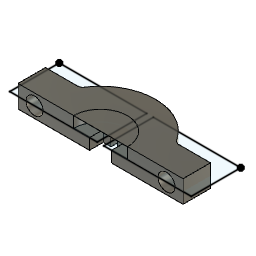
holder_clamp v2 (Autodesk Fusion 360 design; units mm, degrees)
Autodesk Fusion 360 part; units mm, degrees
sketch "スケッチ1" plane through (0, 0, 0) normal (0, 0, 1) x (1, 0, 0)
  line L0 (-16.5, 22) -> (16.5, 22)
  line L1 (16.5, 22) -> (16.5, 0)
  line L2 (16.5, 0) -> (-16.5, 0)
  line L3 (-16.5, 0) -> (-16.5, 22)
  dimension "d7" = 22
  dimension "d8" = 33
  constraint horizontal L0
  constraint vertical L1
  constraint horizontal L2
  constraint vertical L3
  constraint coincident origin L2
  constraint midpoint origin L2
  measures "d7" distance of L0.end L1.end
  measures "d8" distance of L0.start L0.end
extrude "押し出し1" add sketch "スケッチ1" along normal blind 2
sketch "スケッチ3" plane through (0, 0, 0) normal (0, 0, -1) x (1, 0, 0)
  line L0 (16.5, 0) -> (-16.5, 0)
  line L1 (-16.5, 0) -> (-16.5, -22)
  line L2 (-16.5, -22) -> (16.5, -22)
  line L3 (16.5, -22) -> (16.5, 0)
  arc A0 (-4.9, -13) -> (4.9, -13) centre (0, -13) ccw
  line L4 (16.5, -13) -> (-16.5, -13)
  dimension "d9" = 9.8
  dimension "d10" = 9
  constraint coincident L3 L4.start
  constraint coincident L1 L4.end
  constraint perpendicular L1 L4
  constraint coincident A0.centre L4
  measures "d9" diameter of A0
  measures "d10" distance of L2 A0.centre
extrude "押し出し2" add sketch "スケッチ3" along normal blind 2 contours L1 L2 L3 A0 L4
sketch "スケッチ4" plane through (0, 0, -2) normal (0, 0, -1) x (1, 0, 0)
  line L0 (-4.9, -13) -> (-16.5, -13)
  line L1 (-16.5, -13) -> (-16.5, -22)
  line L2 (-16.5, -22) -> (16.5, -22)
  line L3 (16.5, -22) -> (16.5, -13)
  line L4 (16.5, -13) -> (4.9, -13)
  arc A0 (-4.9, -13) -> (4.9, -13) centre (0, -13) ccw
  line L5 (16.5, -22) -> (0.6, -22)
  line L6 (0.6, -22) -> (0.6, -13)
  line L7 (0.6, -13) -> (16.5, -13)
  line L8 (16.5, -13) -> (16.5, -22)
  line L9 (-16.5, -22) -> (-0.6, -22)
  line L10 (-0.6, -22) -> (-0.6, -13)
  line L11 (-0.6, -13) -> (-16.5, -13)
  line L12 (-16.5, -13) -> (-16.5, -22)
  dimension "d13" = 1.2
  constraint horizontal L5
  constraint vertical L6
  constraint horizontal L7
  constraint vertical L8
  constraint coincident L2.end L3.start
  constraint horizontal L9
  constraint vertical L10
  constraint horizontal L11
  constraint vertical L12
  constraint coincident L1.end L2.start
  constraint equal L5 L9
  constraint equal L8 L12
  constraint equal L1 L12
  measures "d13" distance of L6 L10
extrude "押し出し3" add sketch "スケッチ4" along normal blind 2
sketch "スケッチ5" plane through (0, 0, 0) normal (0, 0, -1) x (1, 0, 0)
  line L0 (4.9, -13) -> (16.5, -13)
  line L1 (16.5, -13) -> (16.5, 0)
  line L2 (16.5, 0) -> (-16.5, 0)
  line L3 (-16.5, 0) -> (-16.5, -13)
  line L4 (-16.5, -13) -> (-4.9, -13)
  arc A0 (-4.9, -13) -> (4.9, -13) centre (0, -13) ccw
  line L5 (-3.75, 0) -> (3.75, 0)
  line L6 (3.75, 0) -> (3.75, -18)
  line L7 (3.75, -18) -> (-3.75, -18)
  line L8 (-3.75, -18) -> (-3.75, 0)
  line L9 (0, -1.75) -> (0, -22.5)
  line L10 (3.75, -7) -> (16.5, -7)
  line L11 (-3.75, -7) -> (-16.5, -7)
  dimension "d17" = 7.5
  dimension "d18" = 11
  dimension "d19" = 11
  constraint horizontal L5
  constraint vertical L6
  constraint horizontal L7
  constraint vertical L8
  constraint coincident L2 L5.start
  constraint symmetric L6 L8 L9
  constraint coincident L6 L10.start
  constraint perpendicular L6 L10
  constraint coincident L1 L10.end
  constraint coincident L8 L11.start
  constraint coincident L3 L11.end
  constraint perpendicular L3 L11
  measures "d17" distance of L5.start L5.end
  measures "d18" distance of L6.end L10.start
  measures "d19" distance of L7.end L11.start
sketch "スケッチ9" plane through (0, 13, 0) normal (0, -1, 0) x (1, 0, 0)
  line L0 (-4.9, 0) -> (-16.5, 0)
  line L1 (-16.5, 0) -> (-16.5, -4)
  line L2 (-16.5, -4) -> (-0.6, -4)
  line L3 (-0.6, -4) -> (-0.6, -2)
  line L4 (-0.6, -2) -> (-4.9, -2)
  line L5 (-4.9, -2) -> (-4.9, 0)
  line L6 (-2, -2) -> (2, -2)
  line L7 (2, -2) -> (2, -4)
  line L8 (2, -4) -> (-2, -4)
  line L9 (-2, -4) -> (-2, -2)
  line L10 (16.5, -4) -> (0.6, -4)
  dimension "d37" = 4
  dimension "d38" = 2
  constraint horizontal L6
  constraint vertical L7
  constraint horizontal L8
  constraint vertical L9
  constraint coincident L4 L6.start
  constraint collinear L8 L10
  measures "d37" distance of L7.end L8.end
  measures "d38" distance of origin L7
extrude "押し出し7" cut sketch "スケッチ9" against normal blind 2.5 contours L2 L3 L4 L6 L8 L9 | L3 L6 L7 L8 L10
sketch "スケッチ11" plane through (0, 22, 0) normal (0, 1, 0) x (-1, 0, 0)
  line L0 (16.5, -4) -> (16.5, 2)
  line L1 (16.5, 2) -> (-16.5, 2)
  line L2 (-16.5, 2) -> (-16.5, -4)
  line L3 (-16.5, -4) -> (16.5, -4)
  line L4 (16.5, 2) -> (-13.5, 2)
  line L5 (-13.5, 2) -> (-13.5, 12)
  line L6 (-13.5, 12) -> (16.5, 12)
  line L7 (16.5, 12) -> (16.5, 2)
  dimension "d49" = 10
  constraint horizontal L4
  constraint vertical L5
  constraint horizontal L6
  constraint vertical L7
  constraint coincident L0.end L1.start
  measures "d49" distance of L0.end L6.end
ref_plane "作業平面1" through (0, 11, -1) normal (0, 1, 0) x (-1, 0, 0)
sketch "スケッチ13" plane through (0, 11, -1) normal (0, 1, 0) x (1, 0, 0)
  line L0 (16.5, -10) -> (-16.5, -10)
  line L1 (-16.5, -10) -> (-16.5, -3)
  line L2 (-16.5, -3) -> (16.5, -3)
  line L3 (16.5, -3) -> (16.5, -10)
  line L4 (16.5, 3) -> (16.5, -3)
  line L5 (-16.5, 3) -> (-16.5, -3)
  circle A0 centre (0, -6.5) radius 2.25
  dimension "d53" = 7
  dimension "d54" = 4.5
  dimension "d58" = 3.5
  constraint horizontal L0
  constraint vertical L1
  constraint horizontal L2
  constraint vertical L3
  constraint collinear L3 L4
  constraint coincident L2 L1.end
  measures "d53" distance of L0.end L1.end
  measures "d54" diameter of A0
  measures "d58" distance of L2 A0.centre
extrude "押し出し11" add sketch "スケッチ13" along normal blind -2 and the other way blind -8
sketch "Sketch17" plane through (16.5, 0, 0) normal (1, 0, 0) x (0, 1, 0)
  line L0 (22, -4) -> (22, 2)
  line L1 (22, 2) -> (19, 2)
  line L2 (19, 2) -> (19, 9)
  line L3 (19, 9) -> (9, 9)
  line L4 (9, 9) -> (9, 2)
  line L5 (9, 2) -> (0, 2)
  line L6 (0, 2) -> (0, 0)
  line L7 (0, 0) -> (13, 0)
  line L8 (13, 0) -> (13, -4)
  line L9 (13, -4) -> (22, -4)
  line L10 (11, 9) -> (17, 9)
  line L11 (17, 9) -> (17, 2)
  line L12 (17, 2) -> (11, 2)
  line L13 (11, 2) -> (11, 9)
  constraint horizontal L10
  constraint vertical L11
  constraint horizontal L12
  constraint vertical L13
  constraint coincident L3 L10.start
extrude "Extrude15" cut sketch "Sketch17" against normal blind 400 contours L3 L10 L11 L12 L13
sketch "Sketch18" plane through (-16.5, 0, 0) normal (-1, 0, 0) x (0, -1, 0)
  line L0 (-11, 9) -> (-11, 2)
  line L1 (-11, 2) -> (-17, 2)
  line L2 (-17, 2) -> (-17, 9)
  line L3 (-17, 9) -> (-19, 9)
  line L4 (-19, 9) -> (-19, 2)
  line L5 (-19, 2) -> (-22, 2)
  line L6 (-22, 2) -> (-22, -4)
  line L7 (-22, -4) -> (-13, -4)
  line L8 (-13, -4) -> (-13, 0)
  line L9 (-13, 0) -> (0, 0)
  line L10 (0, 0) -> (0, 2)
  line L11 (0, 2) -> (-9, 2)
  line L12 (-9, 2) -> (-9, 9)
  line L13 (-9, 9) -> (-11, 9)
  line L14 (-9, 2) -> (0, 2)
  line L15 (0, 2) -> (0, 0)
  line L16 (0, 0) -> (-9, 0)
  line L17 (-9, 0) -> (-9, 2)
  constraint horizontal L14
  constraint vertical L15
  constraint horizontal L16
  constraint vertical L17
  constraint coincident L9.end L10.start
  constraint coincident L11.end L12.start
extrude "Extrude16" cut sketch "Sketch18" against normal blind 34 contours L9 L10 L11 L14 L15 L16 L17
sketch "Sketch19" plane through (-16.5, 0, 0) normal (-1, 0, 0) x (0, -1, 0)
  line L0 (-9, 0) -> (-9, 9)
  line L1 (-9, 9) -> (-11, 9)
  line L2 (-11, 9) -> (-11, 2)
  line L3 (-11, 2) -> (-17, 2)
  line L4 (-17, 2) -> (-17, 9)
  line L5 (-17, 9) -> (-19, 9)
  line L6 (-19, 9) -> (-19, 2)
  line L7 (-19, 2) -> (-22, 2)
  line L8 (-22, 2) -> (-22, -4)
  line L9 (-22, -4) -> (-13, -4)
  line L10 (-13, -4) -> (-13, 0)
  line L11 (-13, 0) -> (-9, 0)
  line L12 (-19, 9) -> (-9, 9)
  line L13 (-9, 9) -> (-9, 2)
  line L14 (-9, 2) -> (-19, 2)
  line L15 (-19, 2) -> (-19, 9)
  constraint horizontal L12
  constraint vertical L13
  constraint horizontal L14
  constraint vertical L15
  constraint coincident L0 L13.end
  constraint coincident L5.end L6.start
extrude "Extrude17" cut sketch "Sketch19" against normal blind 34 contours L0 L1 L2 L12 L13 L14 | L2 L3 L4 L12 L14 | L4 L5 L6 L12 L14 L15
sketch "Sketch20" plane through (-16.5, 0, 0) normal (-1, 0, 0) x (0, -1, 0)
  line L0 (-9, 2) -> (-22, 2)
  line L1 (-22, 2) -> (-22, -4)
  line L2 (-22, -4) -> (-13, -4)
  line L3 (-13, -4) -> (-13, 0)
  line L4 (-13, 0) -> (-9, 0)
  line L5 (-9, 0) -> (-9, 2)
  line L6 (-13, 2) -> (-9, 2)
  line L7 (-9, 2) -> (-9, 0)
  line L8 (-9, 0) -> (-13, 0)
  line L9 (-13, 0) -> (-13, 2)
  constraint horizontal L6
  constraint vertical L7
  constraint horizontal L8
  constraint vertical L9
  constraint coincident L4.end L5.start
  constraint coincident L0 L6.start
extrude "Extrude18" cut sketch "Sketch20" against normal blind 3400 contours L0 L4 L5 L6 L7 L8 L9
sketch "Sketch21" plane through (0, 13, 0) normal (0, -1, 0) x (1, 0, 0)
  line L0 (-2, -4) -> (-2, -2)
  line L1 (-2, -2) -> (-4.9, -2)
  line L2 (-4.9, -2) -> (-4.9, 0)
  line L3 (-4.9, 0) -> (4.9, 0)
  line L4 (4.9, 0) -> (4.9, -2)
  line L5 (4.9, -2) -> (2, -2)
  line L6 (2, -2) -> (2, -4)
  line L7 (2, -4) -> (16.5, -4)
  line L8 (16.5, -4) -> (16.5, 2)
  line L9 (16.5, 2) -> (-16.5, 2)
  line L10 (-16.5, 2) -> (-16.5, -4)
  line L11 (-16.5, -4) -> (-2, -4)
  line L12 (-16.5, 2) -> (16.5, 2)
  line L13 (16.5, 2) -> (16.5, 0.0267)
  line L14 (16.5, 0.0267) -> (-16.5, 0.0267)
  line L15 (-16.5, 0.0267) -> (-16.5, 2)
  constraint horizontal L12
  constraint vertical L13
  constraint horizontal L14
  constraint vertical L15
  constraint coincident L8 L13.end
  constraint coincident L9.end L10.start
extrude "Extrude19" cut sketch "Sketch21" against normal blind 15 contours L8 L9 L10 L12 L13 L14 L15
sketch "Sketch22" plane through (0, 0, -4) normal (0, 0, -1) x (1, 0, 0)
  line L0 (2, -13) -> (2, -15.5)
  line L1 (2, -15.5) -> (0.6, -15.5)
  line L2 (0.6, -15.5) -> (0.6, -17.8631)
  arc A0 (-0.6, -17.8631) -> (0.6, -17.8631) centre (0, -13) ccw
  line L3 (-0.6, -17.8631) -> (-0.6, -15.5)
  line L4 (-0.6, -15.5) -> (-2, -15.5)
  line L5 (-2, -15.5) -> (-2, -13)
  line L6 (-2, -13) -> (-16.5, -13)
  line L7 (-16.5, -13) -> (-16.5, -22)
  line L8 (-16.5, -22) -> (16.5, -22)
  line L9 (16.5, -22) -> (16.5, -13)
  line L10 (16.5, -13) -> (2, -13)
  circle A1 centre (0, -13) radius 9.001
  line L11 (-16.5, -13) -> (16.5, -13)
  line L12 (16.5, -13) -> (16.5, -18)
  line L13 (16.5, -18) -> (-16.5, -18)
  line L14 (-16.5, -18) -> (-16.5, -13)
  constraint concentric A0 A1
  constraint horizontal L11
  constraint vertical L12
  constraint horizontal L13
  constraint vertical L14
  constraint coincident L9 L12.end
  constraint coincident L6.end L7.start
extrude "Extrude20" cut sketch "Sketch22" against normal blind 10 contours L8 L9 A1 L13 | L7 L8 A1 L13
move_face "OffsetFaces1" offset -1 1 faces at (16.5, 16.3333, -1.3244)
move_face "OffsetFaces2" offset -0.5 1 faces at (15.5, 16.3333, -1.3244)
move_face "OffsetFaces3" offset -1.5 1 faces at (-16.5, 16.3333, -1.3244)
move_face "OffsetFaces4" offset 1 1 faces at (0.0456, 22, -1.3156)
fillet "Fillet1" radius 1 1 edges at (8.6615, 18, -1.9867)
fillet "Fillet2" radius 1 1 edges at (-8.6615, 18, -1.9867)
sketch "Sketch23" plane through (0, 18, 0) normal (0, 1, 0) x (-1, 0, 0)
  line L0 (9.2208, 0.0267) -> (9.2208, -4)
  line L1 (9.2208, -4) -> (15, -4)
  line L2 (15, -4) -> (15, 0.0267)
  line L3 (15, 0.0267) -> (9.2208, 0.0267)
  point P0 (12, -1.9867)
  point P1 (-12, -2)
hole "Hole1" at (-12, 18, -1.9867) at (12, 18, -2) direction (0, -1, 0) diameter 3.1 depth 10 tip angle 118
